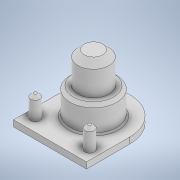
# Autodesk Inventor part: soporte_brazo_art
Saved by Autodesk Inventor 2021 (Build 250183000, 183)
## iProperties
Created: 2021-12-09
Part Number: soporte_brazo_art
Material: Genérico
Document SubType Name: Modeling
Designer: Joaquín
Density: 1 g/cm^3
Appearance: Valor por defecto
Author: Joaquín
Autodesk Inventor part; units mm, degrees
ref_plane "YZ Plane" through (0, 0, 0) normal (1, 0, 0) x (0, 1, 0)
ref_plane "XZ Plane" through (0, 0, 0) normal (0, 1, 0) x (-1, 0, 0)
ref_plane "XY Plane" through (0, 0, 0) normal (0, 0, 1) x (1, 0, 0)
sketch "Boceto1" plane through (0, 0, 0) normal (0, 1, 0) x (-1, 0, 0)
  circle A0 centre (0, 0) radius 8
  circle A1 centre (8.75, 10) radius 1.5
  circle A2 centre (-8.75, 10) radius 1.5
  circle A3 centre (-8.75, 10) radius 1.5
  circle A4 centre (8.75, 10) radius 1.5
  line L0 (11.75, 10) -> (11.75, 14)
  line L1 (11.75, 14) -> (-8.75, 14)
  line L2 (-11.75, 10) -> (-11.75, 14)
  line L3 (-11.75, 14) -> (-8.75, 14)
  arc A5 (-11.75, 0) -> (11.75, 0) centre (0, 0) ccw
  line L4 (11.75, 0) -> (11.75, 10)
  line L5 (-11.75, 0) -> (-11.75, 10.3265)
  constraints: 12 end point, 6 centre point, 3 coincident, 2 perpendicular, 2 point on circle, 2 point on line, 2 vertical, 1 concentric
extrude "Extrusión1" add sketch "Boceto1" along normal blind 3
sketch "Boceto2" plane through (0, 0, 0) normal (0, -1, 0) x (1, 0, 0)
  circle A0 centre (8.75, 10) radius 1.5 projected
  circle A1 centre (8.75, 10) radius 1.5
  circle A2 centre (-8.75, 10) radius 1.5 projected
  circle A3 centre (-8.75, 10) radius 1.5
  point P0 (0, 0)
  constraints: 2 centre point, 2 coincident
extrude "Extrusión2" add sketch "Boceto2" against normal blind 10
sketch "Boceto3" plane through (0, 0, 0) normal (0, -1, 0) x (1, 0, 0)
  circle A0 centre (0, 0) radius 8
  constraints: 1 centre point, 1 coincident
extrude "Extrusión3" add sketch "Boceto3" against normal blind 3.5
sketch "Boceto4" plane through (0, 3.5, 0) normal (0, 1, 0) x (1, 0, 0)
  circle A0 centre (0, 0) radius 7.5
  dimension "d16" = 15
  constraints: 1 centre point, 1 coincident
  measures "d16" diameter of A0
extrude "Extrusión4" add sketch "Boceto4" along normal blind 8
sketch "Boceto5" plane through (0, 11.5, 0) normal (0, 1, 0) x (1, 0, 0)
  circle A0 centre (0, 0) radius 5
  dimension "d19" = 10
  constraints: 1 centre point, 1 coincident
  measures "d19" diameter of A0
extrude "Extrusión5" add sketch "Boceto5" along normal blind 10
chamfer "Chaflán1" distance 0.5 angle 45 1 edges at (-8, 3.5, 0)
chamfer "Chaflán2" distance 1 angle 45 1 edges at (-7.5, 11.5, 0)
chamfer "Chaflán3" distance 2 angle 45 1 edges at (-5, 21.5, 0)
chamfer "Chaflán4" distance 1 angle 45 2 edges at (-10.25, 10, 10) (7.25, 10, 10)
chamfer "Chaflán5" distance 1 angle 45 4 edges at (0, 0, 14) (11.75, 0, 7) (0, 0, -11.75) (-11.75, 0, 7)
